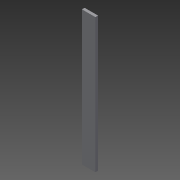
# Autodesk Inventor part: carrier plank long
Saved by Autodesk Inventor 2015 (Build 190159000, 159)
## iProperties
Created: 2019-04-11
Part Number: carrier plank long
Material: Generic
Document SubType Name: Modeling
Designer: Raptor
Density: 1 g/cm^3
Appearance: Default
Author: Raptor
Autodesk Inventor part; units mm, degrees
ref_plane "YZ Plane" through (0, 0, 0) normal (1, 0, 0) x (0, 1, 0)
ref_plane "XZ Plane" through (0, 0, 0) normal (0, 1, 0) x (-1, 0, 0)
ref_plane "XY Plane" through (0, 0, 0) normal (0, 0, 1) x (1, 0, 0)
sketch "Sketch1" plane through (0, 0, 0) normal (0, 1, 0) x (-1, 0, 0)
  line L0 (0, 0) -> (100, 0)
  line L1 (100, 0) -> (100, -1000)
  line L2 (100, -1000) -> (0, -1000)
  line L3 (0, -1000) -> (0, 0)
  dimension "d0" = 1000
  dimension "d1" = 100
  constraints: 8 end point, 2 parallel, 1 horizontal, 1 perpendicular
  measures "d0" distance of L0.end L1.end
  measures "d1" distance of L0.start L0.end
extrude "Extrusion1" add sketch "Sketch1" along normal blind 20
body "Solid1"
